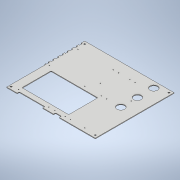
# Autodesk Inventor part: right_pane_inner
Saved by Autodesk Inventor 2022 (Build 260153000, 153)
## iProperties
Created: 2021-05-16
Part Number: right_pane_inner
Material: Generic
Document SubType Name: Modeling
Designer: gisen
Density: 1 g/cm^3
Appearance: Default
Author: gisen
Autodesk Inventor part; units mm, degrees
ref_plane "YZ Plane" through (0, 0, 0) normal (1, 0, 0) x (0, 1, 0)
ref_plane "XZ Plane" through (0, 0, 0) normal (0, 1, 0) x (-1, 0, 0)
ref_plane "XY Plane" through (0, 0, 0) normal (0, 0, 1) x (1, 0, 0)
sketch "Sketch1" plane through (0, 0, 0) normal (0, 0, 1) x (1, 0, 0)
  line L0 (-195, 172) -> (195, 172)
  line L1 (195, 172) -> (195, -172)
  line L2 (195, -172) -> (-195, -172)
  line L3 (-195, -172) -> (-195, 172)
  line L4 (-195, 172) -> (195, -172) construction
  line L5 (195, 172) -> (-195, -172) construction
  point P0 (0, 0)
  dimension "d0" = 390
  dimension "d1" = 344
  constraints: 12 end point, 2 midpoint, 2 parallel, 1 horizontal, 1 perpendicular
  measures "d0" distance of L0.start L0.end
  measures "d1" distance of L0.end L1.end
extrude "Extrusion1" add sketch "Sketch1" along normal blind 3
sketch "Sketch2" plane through (0, 0, 3) normal (0, 0, 1) x (1, 0, 0)
  line L0 (195, 172) -> (-195, 172) projected
  line L1 (-195, 172) -> (-195, -172) projected
  line L2 (-195, -172) -> (195, -172) projected
  line L3 (195, -172) -> (195, 172) projected
  arc A0 (-183.7153, 163.8472) -> (-186.8472, 160.7153) centre (-185, 162) ccw
  arc A1 (-185.2577, 158.4298) -> (-181.4298, 162.2577) centre (-183, 160) ccw
  line L4 (-183.7153, 163.8472) -> (-181.4298, 162.2577)
  line L5 (-186.8472, 160.7153) -> (-185.2577, 158.4298)
  arc A2 (-186.8472, -160.7153) -> (-183.7153, -163.8472) centre (-185, -162) ccw
  arc A3 (-181.4298, -162.2577) -> (-185.2577, -158.4298) centre (-183, -160) ccw
  arc A4 (183.7153, -163.8472) -> (186.8472, -160.7153) centre (185, -162) ccw
  arc A5 (185.2577, -158.4298) -> (181.4298, -162.2577) centre (183, -160) ccw
  arc A6 (186.8472, 160.7153) -> (183.7153, 163.8472) centre (185, 162) ccw
  arc A7 (181.4298, 162.2577) -> (185.2577, 158.4298) centre (183, 160) ccw
  line L6 (183.7153, 163.8472) -> (181.4298, 162.2577)
  line L7 (186.8472, 160.7153) -> (185.2577, 158.4298)
  line L8 (185.2577, -158.4298) -> (186.8472, -160.7153)
  line L9 (181.4298, -162.2577) -> (183.7153, -163.8472)
  line L10 (-185.2577, -158.4298) -> (-186.8511, -160.7209)
  line L11 (-183.7153, -163.8472) -> (-181.4298, -162.2577)
  point P0 (0, 0)
  dimension "d4" = 10
  dimension "d5" = 10
  dimension "d6" = 12
  dimension "d7" = 12
  dimension "d8" = 4.5
  dimension "d9" = 5.5
  dimension "d10" = 12
  dimension "d11" = 12
  dimension "d12" = 10
  dimension "d13" = 10
  dimension "d14" = 10
  dimension "d15" = 10
  dimension "d16" = 12
  dimension "d17" = 12
  dimension "d18" = 12
  dimension "d19" = 12
  dimension "d20" = 10
  dimension "d21" = 10
  dimension "d22" = 4.5
  dimension "d23" = 5.5
  dimension "d24" = 4.5
  dimension "d25" = 5.5
  dimension "d26" = 4.5
  dimension "d27" = 5.5
  constraints: 16 end point, 16 point on circle, 16 tangent, 8 centre point, 8 coincident, 1 point on line
  measures "d4" distance from line of L0 point (-185, 162)
  measures "d5" distance from line of L1 point (-185, 162)
  measures "d6" distance from line of L0 point (-183, 160)
  measures "d7" distance from line of L1 point (-183, 160)
  measures "d8" diameter of A0
  measures "d9" diameter of A1
  measures "d10" distance from line of L0 point (183, 160)
  measures "d11" distance from line of L3 point (183, 160)
  measures "d12" distance from line of L0 point (185, 162)
  measures "d13" distance from line of point (185, 162) L3
  measures "d14" distance from line of L2 point (-185, -162)
  measures "d15" distance from line of L1 point (-185, -162)
  measures "d16" distance from line of L2 point (-183, -160)
  measures "d17" distance from line of L1 point (-183, -160)
  measures "d18" distance from line of L2 point (183, -160)
  measures "d19" distance from line of L3 point (183, -160)
  measures "d20" distance from line of L3 point (185, -162)
  measures "d21" distance from line of L2 point (185, -162)
  measures "d22" diameter of A2
  measures "d23" diameter of A3
  measures "d24" diameter of A4
  measures "d25" diameter of A5
  measures "d26" diameter of A6
  measures "d27" diameter of A7
extrude "Extrusion2" cut sketch "Sketch2" against normal up to surface (3 mm away) contours L4 A1 L5 A0 | L10 A3 L11 A2 | L9 A5 L8 A4 | L7 A7 L6 A6
sketch "Sketch3" plane through (0, 0, 3) normal (0, 0, 1) x (1, 0, 0)
  line L0 (195, 172) -> (-195, 172) projected
  line L1 (-195, 172) -> (-195, -172) projected
  line L2 (-195, -2.564) -> (-191.5, -2.564)
  line L3 (-191.5, -2.564) -> (-191.5, -172)
  line L4 (-191.5, -172) -> (-195, -172)
  line L5 (-195, -172) -> (-195, -2.564)
  line L6 (-195, -2.564) -> (-191.5, -172) construction
  line L7 (-191.5, -2.564) -> (-195, -172) construction
  line L8 (-195, -172) -> (195, -172) projected
  line L9 (-195, -172) -> (-195, 172) projected
  line L10 (-195, 12.893) -> (-190.5, 12.893)
  line L11 (-190.5, 12.893) -> (-190.5, 2.106)
  line L12 (-190.5, 2.106) -> (-195, 2.106)
  line L13 (-195, 2.106) -> (-195, 12.893)
  line L14 (-195, 12.893) -> (-190.5, 2.106) construction
  line L15 (-190.5, 12.893) -> (-195, 2.106) construction
  line L16 (-195, 33.238) -> (-190.5, 33.238)
  line L17 (-190.5, 33.238) -> (-190.5, 22.451)
  line L18 (-190.5, 22.451) -> (-195, 22.451)
  line L19 (-195, 22.451) -> (-195, 33.238)
  line L20 (-195, 33.238) -> (-190.5, 22.451) construction
  line L21 (-190.5, 33.238) -> (-195, 22.451) construction
  line L22 (-195, 53.893) -> (-190.5, 53.893)
  line L23 (-190.5, 53.893) -> (-190.5, 43.106)
  line L24 (-190.5, 43.106) -> (-195, 43.106)
  line L25 (-195, 43.106) -> (-195, 53.893)
  line L26 (-195, 53.893) -> (-190.5, 43.106) construction
  line L27 (-190.5, 53.893) -> (-195, 43.106) construction
  line L28 (-195, 74.238) -> (-190.5, 74.238)
  line L29 (-190.5, 74.238) -> (-190.5, 63.451)
  line L30 (-190.5, 63.451) -> (-195, 63.451)
  line L31 (-195, 63.451) -> (-195, 74.238)
  line L32 (-195, 74.238) -> (-190.5, 63.451) construction
  line L33 (-190.5, 74.238) -> (-195, 63.451) construction
  line L34 (-195, 94.893) -> (-190.5, 94.893)
  line L35 (-190.5, 94.893) -> (-190.5, 84.106)
  line L36 (-190.5, 84.106) -> (-195, 84.106)
  line L37 (-195, 84.106) -> (-195, 94.893)
  line L38 (-195, 94.893) -> (-190.5, 84.106) construction
  line L39 (-190.5, 94.893) -> (-195, 84.106) construction
  line L40 (-195, 115.238) -> (-190.5, 115.238)
  line L41 (-190.5, 115.238) -> (-190.5, 104.451)
  line L42 (-190.5, 104.451) -> (-195, 104.451)
  line L43 (-195, 104.451) -> (-195, 115.238)
  line L44 (-195, 115.238) -> (-190.5, 104.451) construction
  line L45 (-190.5, 115.238) -> (-195, 104.451) construction
  line L46 (-195, 135.893) -> (-190.5, 135.893)
  line L47 (-190.5, 135.893) -> (-190.5, 125.106)
  line L48 (-190.5, 125.106) -> (-195, 125.106)
  line L49 (-195, 125.106) -> (-195, 135.893)
  line L50 (-195, 135.893) -> (-190.5, 125.106) construction
  line L51 (-190.5, 135.893) -> (-195, 125.106) construction
  line L52 (-195, 156.238) -> (-190.5, 156.238)
  line L53 (-190.5, 156.238) -> (-190.5, 145.451)
  line L54 (-190.5, 145.451) -> (-195, 145.451)
  line L55 (-195, 145.451) -> (-195, 156.238)
  line L56 (-195, 156.238) -> (-190.5, 145.451) construction
  line L57 (-190.5, 156.238) -> (-195, 145.451) construction
  point P0 (0, 0)
  point P1 (-193.25, -87.282)
  point P2 (-192.75, 7.4995)
  point P3 (-192.75, 27.8445)
  point P4 (-192.75, 48.4995)
  point P5 (-192.75, 68.8445)
  point P6 (-192.75, 89.4995)
  point P7 (-192.75, 109.8445)
  point P8 (-192.75, 130.4995)
  point P9 (-192.75, 150.8445)
  dimension "d33" = 0
  dimension "d34" = 0
  dimension "d35" = 3.5
  dimension "d36" = 169.436
  dimension "d41" = 4.67
  dimension "d42" = 4.5
  dimension "d43" = 0
  dimension "d44" = 10.787
  dimension "d45" = 9.558
  dimension "d46" = 0
  dimension "d47" = 4.5
  dimension "d48" = 10.787
  dimension "d49" = 9.868
  dimension "d50" = 0
  dimension "d51" = 4.5
  dimension "d52" = 10.787
  dimension "d53" = 9.558
  dimension "d54" = 0
  dimension "d55" = 4.5
  dimension "d56" = 10.787
  dimension "d57" = 9.868
  dimension "d58" = 0
  dimension "d59" = 4.5
  dimension "d60" = 10.787
  dimension "d61" = 9.558
  dimension "d62" = 0
  dimension "d63" = 4.5
  dimension "d64" = 10.787
  dimension "d65" = 9.868
  dimension "d66" = 4.5
  dimension "d67" = 0
  dimension "d68" = 10.787
  dimension "d69" = 4.5
  dimension "d70" = 0
  dimension "d71" = 10.787
  dimension "d72" = 9.558
  constraints: 108 end point, 18 midpoint, 18 parallel, 9 horizontal, 9 perpendicular
  measures "d33" distance between parallel lines of L8 L4
  measures "d34" distance between parallel lines of L1 L5
  measures "d35" distance of L3.end L4.end
  measures "d36" distance of L2.end L3.end
  measures "d41" distance between parallel lines of L2 L12
  measures "d42" distance of L11.end L12.end
  measures "d43" distance between parallel lines of L1 L13
  measures "d44" distance of L10.end L11.end
  measures "d45" distance between parallel lines of L10 L18
  measures "d46" distance between parallel lines of L1 L19
  measures "d47" distance of L16.start L16.end
  measures "d48" distance of L16.end L17.end
  measures "d49" distance between parallel lines of L16 L24
  measures "d50" distance between parallel lines of L25 L9
  measures "d51" distance of L23.end L24.end
  measures "d52" distance of L22.end L23.end
  measures "d53" distance between parallel lines of L22 L30
  measures "d54" distance between parallel lines of L1 L31
  measures "d55" distance of L29.end L30.end
  measures "d56" distance of L28.end L29.end
  measures "d57" distance between parallel lines of L28 L36
  measures "d58" distance between parallel lines of L1 L37
  measures "d59" distance of L35.end L36.end
  measures "d60" distance of L34.end L35.end
  measures "d61" distance between parallel lines of L34 L42
  measures "d62" distance between parallel lines of L43 L1
  measures "d63" distance of L41.end L42.end
  measures "d64" distance of L40.end L41.end
  measures "d65" distance between parallel lines of L40 L48
  measures "d66" distance of L47.end L48.end
  measures "d67" distance between parallel lines of L1 L49
  measures "d68" distance of L46.end L47.end
  measures "d69" distance of L53.end L54.end
  measures "d70" distance between parallel lines of L1 L55
  measures "d71" distance of L52.end L53.end
  measures "d72" distance between parallel lines of L46 L54
extrude "Extrusion3" cut sketch "Sketch3" against normal up to surface (3 mm away)
sketch "Sketch4" plane through (0, 0, 3) normal (0, 0, 1) x (1, 0, 0)
  line L0 (-190.5, 156.238) -> (-190.5, 145.451) projected
  line L1 (-190.5, 135.893) -> (-190.5, 125.106) projected
  line L2 (-190.5, 125.106) -> (-195, 125.106) projected
  line L3 (-190.5, 12.893) -> (-190.5, 2.106) projected
  line L4 (195, 172) -> (-195, 172) projected
  point P0 (0, 0)
  point P1 (-178.988, 126.176)
  point P2 (-178.988, 1.716)
  point P3 (-156.128, -155.764)
  point P4 (-24.0488, 125.676)
  point P5 (-24.0488, 1.216)
  point P6 (-24.048, -156.264)
  point P7 (-1.1888, 125.676)
  point P8 (-1.1888, 46.936)
  point P9 (2.622, -156.264)
  point P10 (48.342, -156.264)
  point P11 (71.202, -156.264)
  point P12 (133.432, -156.264)
  point P13 (48.3412, 1.216)
  point P14 (71.2012, 1.216)
  point P15 (133.4312, 1.216)
  point P16 (133.4312, 46.936)
  point P17 (48.3412, 125.676)
  point P18 (71.2012, 125.676)
  point P19 (133.4312, 130.756)
  dimension "d76" = 11.512
  dimension "d77" = 1.07
  dimension "d78" = 124.46
  dimension "d79" = 11.512
  dimension "d83" = 154.94
  dimension "d84" = 46.324
  dimension "d85" = 124.46
  dimension "d86" = 154.94
  dimension "d87" = 157.48
  dimension "d88" = 132.08
  dimension "d89" = 157.48
  dimension "d90" = 22.86
  dimension "d91" = 78.74
  dimension "d92" = 26.67
  dimension "d93" = 45.72
  dimension "d94" = 22.86
  dimension "d95" = 62.23
  dimension "d96" = 72.39
  dimension "d97" = 22.86
  dimension "d98" = 62.23
  dimension "d99" = 134.62
  dimension "d100" = 49.53
  dimension "d101" = 22.86
  dimension "d102" = 62.23
  dimension "d103" = 5.08
  measures "d76" distance from line of L1 point (-178.988, 126.176)
  measures "d77" distance from line of point (-178.988, 126.176) L2
  measures "d78" distance of point (-178.988, 1.716) point (-178.988, 126.176)
  measures "d79" distance from line of point (-178.988, 1.716) L3
  measures "d83" distance of point (-178.988, 126.176) point (-24.049, 125.676)
  measures "d84" distance from line of L4 point (-24.049, 125.676)
  measures "d85" distance of point (-24.049, 125.676) point (-24.049, 1.216)
  measures "d86" distance of point (-24.049, 1.216) point (-178.988, 1.716)
  measures "d87" distance of point (-24.048, -156.264) point (-24.049, 1.216)
  measures "d88" horizontal distance of point (-24.048, -156.264) point (-156.128, -155.764)
  measures "d89" vertical distance of point (-156.128, -155.764) point (-178.988, 1.716)
  measures "d90" distance of point (-1.189, 125.676) point (-24.049, 125.676)
  measures "d91" distance of point (-1.189, 125.676) point (-1.189, 46.936)
  measures "d92" distance of point (-24.048, -156.264) point (2.622, -156.264)
  measures "d93" distance of point (48.342, -156.264) point (2.622, -156.264)
  measures "d94" distance of point (71.202, -156.264) point (48.342, -156.264)
  measures "d95" distance of point (71.202, -156.264) point (133.432, -156.264)
  measures "d96" distance of point (-24.049, 1.216) point (48.341, 1.216)
  measures "d97" distance of point (48.341, 1.216) point (71.201, 1.216)
  measures "d98" distance of point (71.201, 1.216) point (133.431, 1.216)
  measures "d99" distance of point (-1.189, 46.936) point (133.431, 46.936)
  measures "d100" distance of point (48.341, 125.676) point (-1.189, 125.676)
  measures "d101" distance of point (48.341, 125.676) point (71.201, 125.676)
  measures "d102" horizontal distance of point (71.201, 125.676) point (133.431, 130.756)
  measures "d103" vertical distance of point (71.201, 125.676) point (133.431, 130.756)
hole "Hole1" at (-178.988, 126.176, 3) at (-178.988, 1.716, 3) at (-156.128, -155.764, 3) at (-24.0488, 125.676, 3) at (-24.0488, 1.216, 3) at (-24.048, -156.264, 3) at (-1.1888, 125.676, 3) at (-1.1888, 46.936, 3) at (2.622, -156.264, 3) at (48.342, -156.264, 3) at (71.202, -156.264, 3) at (133.432, -156.264, 3) at (48.3412, 1.216, 3) at (71.2012, 1.216, 3) at (133.4312, 1.216, 3) at (133.4312, 46.936, 3) at (48.3412, 125.676, 3) at (71.2012, 125.676, 3) at (133.4312, 130.756, 3) direction (0, 0, -1) diameter 3.2 end through all
sketch "Sketch5" plane through (0, 0, 3) normal (0, 0, 1) x (1, 0, 0)
  circle A0 centre (71.2012, 125.676) radius 1.6 projected
  circle A1 centre (133.4312, 46.936) radius 1.6 projected
  circle A2 centre (71.2012, 1.216) radius 1.6 projected
  circle A3 centre (133.432, -156.264) radius 1.6 projected
  circle A4 centre (48.342, -156.264) radius 1.6 projected
  circle A5 centre (-1.1888, 46.936) radius 1.6 projected
  circle A6 centre (-24.048, -156.264) radius 1.6 projected
  circle A7 centre (-24.0488, 125.676) radius 1.6 projected
  circle A8 centre (-178.988, 1.716) radius 1.6 projected
  circle A9 centre (-178.988, 126.176) radius 1.6 projected
  circle A10 centre (-156.128, -155.764) radius 1.6 projected
  circle A11 centre (-24.0488, 1.216) radius 1.6 projected
  circle A12 centre (-1.1888, 125.676) radius 1.6 projected
  circle A13 centre (2.622, -156.264) radius 1.6 projected
  circle A14 centre (71.202, -156.264) radius 1.6 projected
  circle A15 centre (48.3412, 1.216) radius 1.6 projected
  circle A16 centre (133.4312, 1.216) radius 1.6 projected
  circle A17 centre (48.3412, 125.676) radius 1.6 projected
  circle A18 centre (133.4312, 130.756) radius 1.6 projected
  line L0 (-190.5, 145.451) -> (-195, 145.451) projected
  line L1 (-195, 145.451) -> (-195, 135.893) projected
  line L2 (-195, 135.893) -> (-190.5, 135.893) projected
  line L3 (-190.5, 135.893) -> (-190.5, 125.106) projected
  line L4 (-190.5, 125.106) -> (-195, 125.106) projected
  line L5 (-195, 125.106) -> (-195, 115.238) projected
  line L6 (-195, 115.238) -> (-190.5, 115.238) projected
  line L7 (-190.5, 115.238) -> (-190.5, 104.451) projected
  line L8 (-190.5, 104.451) -> (-195, 104.451) projected
  line L9 (-195, 104.451) -> (-195, 94.893) projected
  line L10 (-195, 94.893) -> (-190.5, 94.893) projected
  line L11 (-190.5, 94.893) -> (-190.5, 84.106) projected
  line L12 (-190.5, 84.106) -> (-195, 84.106) projected
  line L13 (-195, 84.106) -> (-195, 74.238) projected
  line L14 (-195, 74.238) -> (-190.5, 74.238) projected
  line L15 (-190.5, 74.238) -> (-190.5, 63.451) projected
  line L16 (-190.5, 63.451) -> (-195, 63.451) projected
  line L17 (-195, 63.451) -> (-195, 53.893) projected
  line L18 (-195, 53.893) -> (-190.5, 53.893) projected
  line L19 (-190.5, 53.893) -> (-190.5, 43.106) projected
  line L20 (-190.5, 43.106) -> (-195, 43.106) projected
  line L21 (-195, 43.106) -> (-195, 33.238) projected
  line L22 (-195, 33.238) -> (-190.5, 33.238) projected
  line L23 (-190.5, 33.238) -> (-190.5, 22.451) projected
  line L24 (-190.5, 22.451) -> (-195, 22.451) projected
  line L25 (-195, 22.451) -> (-195, 12.893) projected
  line L26 (-195, 12.893) -> (-190.5, 12.893) projected
  line L27 (-190.5, 12.893) -> (-190.5, 2.106) projected
  line L28 (-190.5, 2.106) -> (-195, 2.106) projected
  line L29 (-195, 2.106) -> (-195, -2.564) projected
  line L30 (-195, -2.564) -> (-191.5, -2.564) projected
  line L31 (-191.5, -2.564) -> (-191.5, -172) projected
  line L32 (-191.5, -172) -> (195, -172) projected
  line L33 (195, -172) -> (195, 172) projected
  line L34 (195, 172) -> (-195, 172) projected
  line L35 (-195, 172) -> (-195, 156.238) projected
  line L36 (-195, 156.238) -> (-190.5, 156.238) projected
  line L37 (-190.5, 156.238) -> (-190.5, 145.451) projected
  line L38 (185.2577, -158.4298) -> (186.8472, -160.7153) projected
  arc A19 (183.7153, -163.8472) -> (186.8472, -160.7153) centre (185, -162) ccw projected
  line L39 (183.7153, -163.8472) -> (181.4298, -162.2577) projected
  arc A20 (185.2577, -158.4298) -> (181.4298, -162.2577) centre (183, -160) ccw projected
  line L40 (-181.4298, -162.2577) -> (-183.7153, -163.8472) projected
  arc A21 (-186.8472, -160.7153) -> (-183.7153, -163.8472) centre (-185, -162) ccw projected
  line L41 (-186.8472, -160.7153) -> (-185.2577, -158.4298) projected
  arc A22 (-181.4298, -162.2577) -> (-185.2577, -158.4298) centre (-183, -160) ccw projected
  line L42 (181.4298, 162.2577) -> (183.7153, 163.8472) projected
  arc A23 (186.8472, 160.7153) -> (183.7153, 163.8472) centre (185, 162) ccw projected
  line L43 (186.8472, 160.7153) -> (185.2577, 158.4298) projected
  arc A24 (181.4298, 162.2577) -> (185.2577, 158.4298) centre (183, 160) ccw projected
  arc A25 (-183.7153, 163.8472) -> (-186.8472, 160.7153) centre (-185, 162) ccw projected
  line L44 (-183.7153, 163.8472) -> (-181.4298, 162.2577) projected
  arc A26 (-185.2577, 158.4298) -> (-181.4298, 162.2577) centre (-183, 160) ccw projected
  line L45 (-185.2577, 158.4298) -> (-186.8472, 160.7153) projected
  circle A27 centre (133.4312, 1.216) radius 16.5
  circle A28 centre (133.432, 145.201) radius 16.5
  circle A29 centre (133.432, 73.988) radius 16.5
  line L46 (-155.988, -13.784) -> (48.2012, -13.784)
  line L47 (48.2012, -13.784) -> (48.2012, -141.264)
  line L48 (48.2012, -141.264) -> (-155.988, -141.264)
  line L49 (-155.988, -141.264) -> (-155.988, -13.784)
  point P0 (0, 0)
  dimension "d111" = 33
  dimension "d112" = 33
  dimension "d113" = 33
  dimension "d120" = 23
  dimension "d121" = 15
  dimension "d122" = 15
  dimension "d123" = 23
  constraints: 8 end point, 3 centre point, 2 parallel, 1 coincident, 1 horizontal, 1 perpendicular
  measures "d111" diameter of A27
  measures "d112" diameter of A28
  measures "d113" diameter of A29
  measures "d120" distance from line of A8.centre L49
  measures "d121" distance from line of A11.centre L46
  measures "d122" distance from line of L48 A6.centre
  measures "d123" distance from line of A2.centre L47
extrude "Extrusion5" cut sketch "Sketch5" against normal blind 10 contours A27 | A28 | A29 | L46 L47 L48 L49
sketch "Sketch6" plane through (0, 0, 3) normal (0, 0, 1) x (1, 0, 0)
  line L0 (-191.5, -172) -> (195, -172) projected
  circle A0 centre (-24.048, -156.264) radius 1.6 projected
  line L1 (195, 172) -> (-195, 172) projected
  circle A1 centre (-24.0488, 125.676) radius 1.6 projected
  line L2 (-146.128, -172) -> (-34.048, -172)
  line L3 (-34.048, -172) -> (-34.048, -162.764)
  line L4 (-34.048, -162.764) -> (-146.128, -162.764)
  line L5 (-146.128, -162.764) -> (-146.128, -172)
  circle A2 centre (-156.128, -155.764) radius 1.6 projected
  line L6 (12.622, -172) -> (38.342, -172)
  line L7 (38.342, -172) -> (38.342, -162.764)
  line L8 (38.342, -162.764) -> (12.622, -162.764)
  line L9 (12.622, -162.764) -> (12.622, -172)
  circle A3 centre (2.622, -156.264) radius 1.6 projected
  circle A4 centre (48.342, -156.264) radius 1.6 projected
  point P0 (0, 0)
  dimension "d124" = 6.5
  dimension "d125" = 10
  dimension "d126" = 10
  dimension "d127" = 10
  dimension "d128" = 10
  dimension "d129" = 6.5
  constraints: 16 end point, 4 parallel, 2 horizontal, 2 perpendicular, 2 point on line
  measures "d124" distance from line of A0.centre L4
  measures "d125" distance from line of A0.centre L3
  measures "d126" distance from line of A2.centre L5
  measures "d127" distance from line of A3.centre L9
  measures "d128" distance from line of A4.centre L7
  measures "d129" distance from line of A3.centre L8
extrude "Extrusion6" cut sketch "Sketch6" against normal up to surface (3 mm away) contours L5 L4 L3 L0 | L9 L8 L7 L0
fillet "Fillet1" radius 3 8 edges at (-155.988, -13.784, 1.5) (-155.988, -141.264, 1.5) (48.2012, -141.264, 1.5) (48.2012, -13.784, 1.5) (38.342, -162.764, 1.5) (12.622, -162.764, 1.5) (-34.048, -162.764, 1.5) (-146.128, -162.764, 1.5)
equation "\"d14\" = d5"
equation "\"d15\" = d4"
equation "\"d16\" = d7"
equation "\"d17\" = d6"
equation "\"d18\" = d16"
equation "\"d19\" = d17"
equation "\"d20\" = d15"
equation "\"d21\" = d14"
equation "\"d47\" = d42"
equation "\"d48\" = d44"
equation "\"d51\" = d47"
equation "\"d52\" = d48"
equation "\"d55\" = d51"
equation "\"d56\" = d52"
equation "\"d59\" = d55"
equation "\"d60\" = d56"
equation "\"d63\" = d59"
equation "\"d64\" = d60"
equation "\"d66\" = d63"
equation "\"d68\" = d64"
equation "\"d69\" = d66"
equation "\"d71\" = d68"
equation "\"d79\" = d76"
equation "\"d89\" = d87"
equation "\"d127\" = d125"
equation "\"d128\" = d127"
equation "\"d129\" = d124"
body "Solid1"
